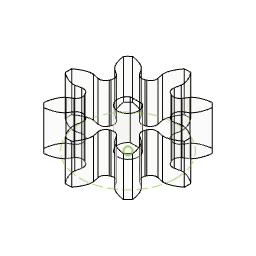
base driver spur gear v1 (Autodesk Fusion 360 archive; units mm, degrees)
design "base driver spur gear" references "Nema 17 groot", "Global Parameters"
description: Spur Gear; Module: 3.0; Num Teeth: 8; Pressure Angle: 20.0; Backlash: 0.00 mm
Autodesk Fusion 360 part; units mm, degrees
imported_body "Derived Base Feature1" makes body 1
other "Derived from Global Parameters v5"
sketch "Sketch1" plane through (0, 0, 0) normal (0, 0, 1) x (1, 0, 0) in component "Spur Gear (8 teeth)"
  circle A0 centre (0, 0) radius 8.3492
extrude "Extrude1" add sketch "Sketch1" along normal blind 10 separate body makes body 2 in component "Spur Gear (8 teeth)"
sketch "Sketch2" plane through (0, 0, 0) normal (0, 0, 1) x (1, 0, 0) in component "Spur Gear (8 teeth)"
  spline S0 degree 5 poles (11.0256, -2.3645) (11.0366, -2.3668) (11.0587, -2.3711) (11.092, -2.3763) (11.1367, -2.3808) (11.193, -2.3832) (11.2496, -2.3833) (11.3065, -2.3819) (11.3634, -2.3798) (11.4205, -2.3772) (11.4776, -2.3739) (11.5348, -2.3698) (11.5921, -2.3647) (11.6496, -2.3584) (11.7071, -2.3509) (11.7647, -2.3424) (11.8223, -2.3329) (11.88, -2.3226) (11.9378, -2.3117) (11.9955, -2.3) (12.0533, -2.2877) (12.111, -2.2747) (12.1688, -2.261) (12.2266, -2.2464) (12.2844, -2.2311) (12.3422, -2.2151) (12.4, -2.1984) (12.4578, -2.181) (12.5155, -2.163) (12.5732, -2.1444) (12.6309, -2.1252) (12.6886, -2.1053) (12.7462, -2.0848) (12.8038, -2.0636) (12.8613, -2.0419) (12.9188, -2.0195) (12.9762, -1.9965) (13.0336, -1.9729) (13.0909, -1.9488) (13.1481, -1.9241) (13.2052, -1.8988) (13.2623, -1.8729) (13.3193, -1.8465) (13.3763, -1.8195) (13.4331, -1.792) (13.4899, -1.7639) (13.5466, -1.7353) (13.6031, -1.7061) (13.6596, -1.6764) (13.716, -1.6461) (13.7723, -1.6153) (13.8284, -1.584) (13.8845, -1.5522) (13.9404, -1.5199) (13.9963, -1.487) (14.052, -1.4537) (14.1076, -1.4198) (14.163, -1.3854) (14.2183, -1.3506) (14.2735, -1.3152) (14.3286, -1.2793) (14.3836, -1.243) (14.4384, -1.2061) (14.493, -1.1688) (14.5475, -1.131) (14.6019, -1.0927) (14.6561, -1.054) (14.7102, -1.0147) (14.7641, -0.975) (14.8178, -0.9349) (14.8714, -0.8943) (14.9141, -0.8614) (14.9461, -0.8365) (14.9674, -0.8198) (14.978, -0.8115) knots 0 0 0 0 0 0 0.01428571 0.02857143 0.04285714 0.05714286 0.07142857 0.08571429 0.1 0.11428571 0.12857143 0.14285714 0.15714286 0.17142857 0.18571429 0.2 0.21428571 0.22857143 0.24285714 0.25714286 0.27142857 0.28571429 0.3 0.31428571 0.32857143 0.34285714 0.35714286 0.37142857 0.38571429 0.4 0.41428571 0.42857143 0.44285714 0.45714286 0.47142857 0.48571429 0.5 0.51428571 0.52857143 0.54285714 0.55714286 0.57142857 0.58571429 0.6 0.61428571 0.62857143 0.64285714 0.65714286 0.67142857 0.68571429 0.7 0.71428571 0.72857143 0.74285714 0.75714286 0.77142857 0.78571429 0.8 0.81428571 0.82857143 0.84285714 0.85714286 0.87142857 0.88571429 0.9 0.91428571 0.92857143 0.94285714 0.95714286 0.97142857 0.98571429 1 1 1 1 1 1
  spline S1 degree 5 poles (11.0256, 2.3645) (11.0366, 2.3668) (11.0587, 2.3711) (11.092, 2.3763) (11.1367, 2.3808) (11.193, 2.3832) (11.2496, 2.3833) (11.3065, 2.3819) (11.3634, 2.3798) (11.4205, 2.3772) (11.4776, 2.3739) (11.5348, 2.3698) (11.5921, 2.3647) (11.6496, 2.3584) (11.7071, 2.3509) (11.7647, 2.3424) (11.8223, 2.3329) (11.88, 2.3226) (11.9378, 2.3117) (11.9955, 2.3) (12.0533, 2.2877) (12.111, 2.2747) (12.1688, 2.261) (12.2266, 2.2464) (12.2844, 2.2311) (12.3422, 2.2151) (12.4, 2.1984) (12.4578, 2.181) (12.5155, 2.163) (12.5732, 2.1444) (12.6309, 2.1252) (12.6886, 2.1053) (12.7462, 2.0848) (12.8038, 2.0636) (12.8613, 2.0419) (12.9188, 2.0195) (12.9762, 1.9965) (13.0336, 1.9729) (13.0909, 1.9488) (13.1481, 1.9241) (13.2052, 1.8988) (13.2623, 1.8729) (13.3193, 1.8465) (13.3763, 1.8195) (13.4331, 1.792) (13.4899, 1.7639) (13.5466, 1.7353) (13.6031, 1.7061) (13.6596, 1.6764) (13.716, 1.6461) (13.7723, 1.6153) (13.8284, 1.584) (13.8845, 1.5522) (13.9404, 1.5199) (13.9963, 1.487) (14.052, 1.4537) (14.1076, 1.4198) (14.163, 1.3854) (14.2183, 1.3506) (14.2735, 1.3152) (14.3286, 1.2793) (14.3836, 1.243) (14.4384, 1.2061) (14.493, 1.1688) (14.5475, 1.131) (14.6019, 1.0927) (14.6561, 1.054) (14.7102, 1.0147) (14.7641, 0.975) (14.8178, 0.9349) (14.8714, 0.8943) (14.9141, 0.8614) (14.9461, 0.8365) (14.9674, 0.8198) (14.978, 0.8115) knots 0 0 0 0 0 0 0.01428571 0.02857143 0.04285714 0.05714286 0.07142857 0.08571429 0.1 0.11428571 0.12857143 0.14285714 0.15714286 0.17142857 0.18571429 0.2 0.21428571 0.22857143 0.24285714 0.25714286 0.27142857 0.28571429 0.3 0.31428571 0.32857143 0.34285714 0.35714286 0.37142857 0.38571429 0.4 0.41428571 0.42857143 0.44285714 0.45714286 0.47142857 0.48571429 0.5 0.51428571 0.52857143 0.54285714 0.55714286 0.57142857 0.58571429 0.6 0.61428571 0.62857143 0.64285714 0.65714286 0.67142857 0.68571429 0.7 0.71428571 0.72857143 0.74285714 0.75714286 0.77142857 0.78571429 0.8 0.81428571 0.82857143 0.84285714 0.85714286 0.87142857 0.88571429 0.9 0.91428571 0.92857143 0.94285714 0.95714286 0.97142857 0.98571429 1 1 1 1 1 1
  arc A0 (14.978, -0.8115) -> (14.978, 0.8115) centre (0, 0) ccw
  line L0 (8.1538, -1.7507) -> (11.0256, -2.3645)
  line L1 (8.1538, 1.7507) -> (11.0256, 2.3645)
  line L2 (8.1538, -1.7507) -> (8.1538, 1.7507)
  point P0 (11.2938, -2.3821)
  point P1 (11.5687, -2.3667)
  point P2 (11.8476, -2.3283)
  point P3 (12.1296, -2.2702)
  point P4 (12.4138, -2.1942)
  point P5 (12.6995, -2.1013)
  point P6 (12.9862, -1.9923)
  point P7 (13.2734, -1.8677)
  point P8 (13.5605, -1.728)
  point P9 (13.847, -1.5734)
  point P10 (14.1325, -1.4043)
  point P11 (14.4164, -1.2208)
  point P12 (14.6985, -1.0231)
  point P13 (11.2938, 2.3821)
  point P14 (11.5687, 2.3667)
  point P15 (11.8476, 2.3283)
  point P16 (12.1296, 2.2702)
  point P17 (12.4138, 2.1942)
  point P18 (12.6995, 2.1013)
  point P19 (12.9862, 1.9923)
  point P20 (13.2734, 1.8677)
  point P21 (13.5605, 1.728)
  point P22 (13.847, 1.5734)
  point P23 (14.1325, 1.4043)
  point P24 (14.4164, 1.2208)
  point P25 (14.6985, 1.0231)
extrude "Extrude2" add sketch "Sketch2" along normal blind 10 bodies 2 in component "Spur Gear (8 teeth)"
fillet "Fillet1" radius 1.5875 2 edges at (8.1632, -1.7527, 5) (8.1632, 1.7527, 5) on bodies 2 in component "Spur Gear (8 teeth)"
pattern_circular "C-Pattern1" count 8 over 360 about axis through (0, 0, 0) along (0, 0, 1) of "Extrude2", "Fillet1" in component "Spur Gear (8 teeth)"
sketch "Sketch3" plane through (0, 0, 0) normal (0, 0, 1) x (1, 0, 0) in component "Spur Gear (8 teeth)"
  circle A0 centre (0, 0) radius 12 construction
  dimension "dia_spurgear_2" = 24
  measures "dia_spurgear_2" diameter of A0
other "ExternalDerived2"
move_body "Move1" bodies 1 to x (1, 0, 0) y (0, 1, 0) z (0, 0, 1) at (0, 0, -20)
sketch "Sketch1 (2)" plane through (0, 0, 10) normal (0, 0, 1) x (-1, 0, 0)
  arc A0 (-7.6452, 3.3555) -> (-7.7787, 3.0333) centre (0, 0) ccw
  arc A1 (-9.5895, 2.0576) -> (-7.7787, 3.0333) centre (-9.2577, 3.61) ccw
  line L0 (-9.5895, 2.0576) -> (-11.0256, 2.3645)
  spline S0 degree 5 poles (-11.0256, 2.3645) (-11.0366, 2.3668) (-11.0587, 2.3711) (-11.092, 2.3763) (-11.1367, 2.3808) (-11.193, 2.3832) (-11.2496, 2.3833) (-11.3065, 2.3819) (-11.3634, 2.3798) (-11.4205, 2.3772) (-11.4776, 2.3739) (-11.5348, 2.3698) (-11.5921, 2.3647) (-11.6496, 2.3584) (-11.7071, 2.3509) (-11.7647, 2.3424) (-11.8223, 2.3329) (-11.88, 2.3226) (-11.9378, 2.3117) (-11.9955, 2.3) (-12.0533, 2.2877) (-12.111, 2.2747) (-12.1688, 2.261) (-12.2266, 2.2464) (-12.2844, 2.2311) (-12.3422, 2.2151) (-12.4, 2.1984) (-12.4578, 2.181) (-12.5155, 2.163) (-12.5732, 2.1444) (-12.6309, 2.1252) (-12.6886, 2.1053) (-12.7462, 2.0848) (-12.8038, 2.0636) (-12.8613, 2.0419) (-12.9188, 2.0195) (-12.9762, 1.9965) (-13.0336, 1.9729) (-13.0909, 1.9488) (-13.1481, 1.9241) (-13.2052, 1.8988) (-13.2623, 1.8729) (-13.3193, 1.8465) (-13.3763, 1.8195) (-13.4331, 1.792) (-13.4899, 1.7639) (-13.5466, 1.7353) (-13.6031, 1.7061) (-13.6596, 1.6764) (-13.716, 1.6461) (-13.7723, 1.6153) (-13.8284, 1.584) (-13.8845, 1.5522) (-13.9404, 1.5199) (-13.9963, 1.487) (-14.052, 1.4537) (-14.1076, 1.4198) (-14.163, 1.3854) (-14.2183, 1.3506) (-14.2735, 1.3152) (-14.3286, 1.2793) (-14.3836, 1.243) (-14.4384, 1.2061) (-14.493, 1.1688) (-14.5475, 1.131) (-14.6019, 1.0927) (-14.6561, 1.054) (-14.7102, 1.0147) (-14.7641, 0.975) (-14.8178, 0.9349) (-14.8714, 0.8943) (-14.9141, 0.8614) (-14.9461, 0.8365) (-14.9674, 0.8198) (-14.978, 0.8115) knots 0 0 0 0 0 0 0.01428571 0.02857143 0.04285714 0.05714286 0.07142857 0.08571429 0.1 0.11428571 0.12857143 0.14285714 0.15714286 0.17142857 0.18571429 0.2 0.21428571 0.22857143 0.24285714 0.25714286 0.27142857 0.28571429 0.3 0.31428571 0.32857143 0.34285714 0.35714286 0.37142857 0.38571429 0.4 0.41428571 0.42857143 0.44285714 0.45714286 0.47142857 0.48571429 0.5 0.51428571 0.52857143 0.54285714 0.55714286 0.57142857 0.58571429 0.6 0.61428571 0.62857143 0.64285714 0.65714286 0.67142857 0.68571429 0.7 0.71428571 0.72857143 0.74285714 0.75714286 0.77142857 0.78571429 0.8 0.81428571 0.82857143 0.84285714 0.85714286 0.87142857 0.88571429 0.9 0.91428571 0.92857143 0.94285714 0.95714286 0.97142857 0.98571429 1 1 1 1 1 1
  arc A2 (-14.978, 0.8115) -> (-14.978, -0.8115) centre (0, 0) ccw
  spline S1 degree 5 poles (-14.978, -0.8115) (-14.9674, -0.8198) (-14.9461, -0.8365) (-14.9141, -0.8614) (-14.8714, -0.8943) (-14.8178, -0.9349) (-14.7641, -0.975) (-14.7102, -1.0147) (-14.6561, -1.054) (-14.6019, -1.0927) (-14.5475, -1.131) (-14.493, -1.1688) (-14.4384, -1.2061) (-14.3836, -1.243) (-14.3286, -1.2793) (-14.2735, -1.3152) (-14.2183, -1.3506) (-14.163, -1.3854) (-14.1076, -1.4198) (-14.052, -1.4537) (-13.9963, -1.487) (-13.9404, -1.5199) (-13.8845, -1.5522) (-13.8284, -1.584) (-13.7723, -1.6153) (-13.716, -1.6461) (-13.6596, -1.6764) (-13.6031, -1.7061) (-13.5466, -1.7353) (-13.4899, -1.7639) (-13.4331, -1.792) (-13.3763, -1.8195) (-13.3193, -1.8465) (-13.2623, -1.8729) (-13.2052, -1.8988) (-13.1481, -1.9241) (-13.0909, -1.9488) (-13.0336, -1.9729) (-12.9762, -1.9965) (-12.9188, -2.0195) (-12.8613, -2.0419) (-12.8038, -2.0636) (-12.7462, -2.0848) (-12.6886, -2.1053) (-12.6309, -2.1252) (-12.5732, -2.1444) (-12.5155, -2.163) (-12.4578, -2.181) (-12.4, -2.1984) (-12.3422, -2.2151) (-12.2844, -2.2311) (-12.2266, -2.2464) (-12.1688, -2.261) (-12.111, -2.2747) (-12.0533, -2.2877) (-11.9955, -2.3) (-11.9378, -2.3117) (-11.88, -2.3226) (-11.8223, -2.3329) (-11.7647, -2.3424) (-11.7071, -2.3509) (-11.6496, -2.3584) (-11.5921, -2.3647) (-11.5348, -2.3698) (-11.4776, -2.3739) (-11.4205, -2.3772) (-11.3634, -2.3798) (-11.3065, -2.3819) (-11.2496, -2.3833) (-11.193, -2.3832) (-11.1367, -2.3808) (-11.092, -2.3763) (-11.0587, -2.3711) (-11.0366, -2.3668) (-11.0256, -2.3645) knots -1 -1 -1 -1 -1 -1 -0.98571429 -0.97142857 -0.95714286 -0.94285714 -0.92857143 -0.91428571 -0.9 -0.88571429 -0.87142857 -0.85714286 -0.84285714 -0.82857143 -0.81428571 -0.8 -0.78571429 -0.77142857 -0.75714286 -0.74285714 -0.72857143 -0.71428571 -0.7 -0.68571429 -0.67142857 -0.65714286 -0.64285714 -0.62857143 -0.61428571 -0.6 -0.58571429 -0.57142857 -0.55714286 -0.54285714 -0.52857143 -0.51428571 -0.5 -0.48571429 -0.47142857 -0.45714286 -0.44285714 -0.42857143 -0.41428571 -0.4 -0.38571429 -0.37142857 -0.35714286 -0.34285714 -0.32857143 -0.31428571 -0.3 -0.28571429 -0.27142857 -0.25714286 -0.24285714 -0.22857143 -0.21428571 -0.2 -0.18571429 -0.17142857 -0.15714286 -0.14285714 -0.12857143 -0.11428571 -0.1 -0.08571429 -0.07142857 -0.05714286 -0.04285714 -0.02857143 -0.01428571 0 0 0 0 0 0
  line L1 (-11.0256, -2.3645) -> (-9.5895, -2.0576)
  arc A3 (-7.7787, -3.0333) -> (-9.5895, -2.0576) centre (-9.2577, -3.61) ccw
  arc A4 (-8.2357, -5.3259) -> (-7.6452, -3.3555) centre (-9.0989, -3.9936) ccw
  line L2 (-8.2357, -5.3259) -> (-9.4682, -6.1244)
  spline S2 degree 5 poles (-9.4682, -6.1244) (-9.4777, -6.1305) (-9.4963, -6.1431) (-9.5235, -6.1629) (-9.5583, -6.1913) (-9.5998, -6.2295) (-9.6399, -6.2695) (-9.6792, -6.3106) (-9.718, -6.3524) (-9.7564, -6.3946) (-9.7945, -6.4373) (-9.8321, -6.4806) (-9.869, -6.5248) (-9.9051, -6.5698) (-9.9405, -6.6158) (-9.9752, -6.6626) (-10.0092, -6.7101) (-10.0428, -6.7581) (-10.0759, -6.8067) (-10.1085, -6.8557) (-10.1406, -6.9053) (-10.1723, -6.9553) (-10.2034, -7.0059) (-10.234, -7.0571) (-10.264, -7.1088) (-10.2936, -7.1609) (-10.3226, -7.2136) (-10.3512, -7.2667) (-10.3793, -7.3203) (-10.407, -7.3743) (-10.4341, -7.4287) (-10.4608, -7.4835) (-10.4871, -7.5388) (-10.5128, -7.5944) (-10.5381, -7.6505) (-10.5629, -7.707) (-10.5873, -7.7638) (-10.6112, -7.821) (-10.6346, -7.8786) (-10.6576, -7.9366) (-10.6802, -7.9949) (-10.7023, -8.0535) (-10.7239, -8.1125) (-10.7451, -8.1719) (-10.7658, -8.2315) (-10.7861, -8.2915) (-10.8059, -8.3519) (-10.8252, -8.4125) (-10.8442, -8.4734) (-10.8626, -8.5347) (-10.8807, -8.5962) (-10.8983, -8.6581) (-10.9154, -8.7202) (-10.9321, -8.7826) (-10.9483, -8.8454) (-10.9641, -8.9083) (-10.9795, -8.9716) (-10.9944, -9.0351) (-11.0089, -9.0989) (-11.0229, -9.1629) (-11.0365, -9.2272) (-11.0496, -9.2918) (-11.0623, -9.3566) (-11.0746, -9.4216) (-11.0864, -9.4869) (-11.0978, -9.5524) (-11.1087, -9.6182) (-11.1192, -9.6841) (-11.1292, -9.7503) (-11.1388, -9.8167) (-11.148, -9.8833) (-11.155, -9.9368) (-11.16, -9.977) (-11.1633, -10.0038) (-11.1649, -10.0173) knots 0 0 0 0 0 0 0.01428571 0.02857143 0.04285714 0.05714286 0.07142857 0.08571429 0.1 0.11428571 0.12857143 0.14285714 0.15714286 0.17142857 0.18571429 0.2 0.21428571 0.22857143 0.24285714 0.25714286 0.27142857 0.28571429 0.3 0.31428571 0.32857143 0.34285714 0.35714286 0.37142857 0.38571429 0.4 0.41428571 0.42857143 0.44285714 0.45714286 0.47142857 0.48571429 0.5 0.51428571 0.52857143 0.54285714 0.55714286 0.57142857 0.58571429 0.6 0.61428571 0.62857143 0.64285714 0.65714286 0.67142857 0.68571429 0.7 0.71428571 0.72857143 0.74285714 0.75714286 0.77142857 0.78571429 0.8 0.81428571 0.82857143 0.84285714 0.85714286 0.87142857 0.88571429 0.9 0.91428571 0.92857143 0.94285714 0.95714286 0.97142857 0.98571429 1 1 1 1 1 1
  arc A5 (-11.1649, -10.0173) -> (-10.0173, -11.1649) centre (0, 0) ccw
  spline S3 degree 5 poles (-10.0173, -11.1649) (-10.0038, -11.1633) (-9.977, -11.16) (-9.9368, -11.155) (-9.8833, -11.148) (-9.8167, -11.1388) (-9.7503, -11.1292) (-9.6841, -11.1192) (-9.6182, -11.1087) (-9.5524, -11.0978) (-9.4869, -11.0864) (-9.4216, -11.0746) (-9.3566, -11.0623) (-9.2918, -11.0496) (-9.2272, -11.0365) (-9.1629, -11.0229) (-9.0989, -11.0089) (-9.0351, -10.9944) (-8.9716, -10.9795) (-8.9083, -10.9641) (-8.8454, -10.9483) (-8.7826, -10.9321) (-8.7202, -10.9154) (-8.6581, -10.8983) (-8.5962, -10.8807) (-8.5347, -10.8626) (-8.4734, -10.8442) (-8.4125, -10.8252) (-8.3519, -10.8059) (-8.2915, -10.7861) (-8.2315, -10.7658) (-8.1719, -10.7451) (-8.1125, -10.7239) (-8.0535, -10.7023) (-7.9949, -10.6802) (-7.9366, -10.6576) (-7.8786, -10.6346) (-7.821, -10.6112) (-7.7638, -10.5873) (-7.707, -10.5629) (-7.6505, -10.5381) (-7.5944, -10.5128) (-7.5388, -10.4871) (-7.4835, -10.4608) (-7.4287, -10.4341) (-7.3743, -10.407) (-7.3203, -10.3793) (-7.2667, -10.3512) (-7.2136, -10.3226) (-7.1609, -10.2936) (-7.1088, -10.264) (-7.0571, -10.234) (-7.0059, -10.2034) (-6.9553, -10.1723) (-6.9053, -10.1406) (-6.8557, -10.1085) (-6.8067, -10.0759) (-6.7581, -10.0428) (-6.7101, -10.0092) (-6.6626, -9.9752) (-6.6158, -9.9405) (-6.5698, -9.9051) (-6.5248, -9.869) (-6.4806, -9.8321) (-6.4373, -9.7945) (-6.3946, -9.7564) (-6.3524, -9.718) (-6.3106, -9.6792) (-6.2695, -9.6399) (-6.2295, -9.5998) (-6.1913, -9.5583) (-6.1629, -9.5235) (-6.1431, -9.4963) (-6.1305, -9.4777) (-6.1244, -9.4682) knots -1 -1 -1 -1 -1 -1 -0.98571429 -0.97142857 -0.95714286 -0.94285714 -0.92857143 -0.91428571 -0.9 -0.88571429 -0.87142857 -0.85714286 -0.84285714 -0.82857143 -0.81428571 -0.8 -0.78571429 -0.77142857 -0.75714286 -0.74285714 -0.72857143 -0.71428571 -0.7 -0.68571429 -0.67142857 -0.65714286 -0.64285714 -0.62857143 -0.61428571 -0.6 -0.58571429 -0.57142857 -0.55714286 -0.54285714 -0.52857143 -0.51428571 -0.5 -0.48571429 -0.47142857 -0.45714286 -0.44285714 -0.42857143 -0.41428571 -0.4 -0.38571429 -0.37142857 -0.35714286 -0.34285714 -0.32857143 -0.31428571 -0.3 -0.28571429 -0.27142857 -0.25714286 -0.24285714 -0.22857143 -0.21428571 -0.2 -0.18571429 -0.17142857 -0.15714286 -0.14285714 -0.12857143 -0.11428571 -0.1 -0.08571429 -0.07142857 -0.05714286 -0.04285714 -0.02857143 -0.01428571 0 0 0 0 0 0
  line L3 (-6.1244, -9.4682) -> (-5.3259, -8.2357)
  arc A6 (-3.3555, -7.6452) -> (-5.3259, -8.2357) centre (-3.9936, -9.0989) ccw
  arc A7 (-2.0576, -9.5895) -> (-3.0333, -7.7787) centre (-3.61, -9.2577) ccw
  line L4 (-2.0576, -9.5895) -> (-2.3645, -11.0256)
  spline S4 degree 5 poles (-2.3645, -11.0256) (-2.3668, -11.0366) (-2.3711, -11.0587) (-2.3763, -11.092) (-2.3808, -11.1367) (-2.3832, -11.193) (-2.3833, -11.2496) (-2.3819, -11.3065) (-2.3798, -11.3634) (-2.3772, -11.4205) (-2.3739, -11.4776) (-2.3698, -11.5348) (-2.3647, -11.5921) (-2.3584, -11.6496) (-2.3509, -11.7071) (-2.3424, -11.7647) (-2.3329, -11.8223) (-2.3226, -11.88) (-2.3117, -11.9378) (-2.3, -11.9955) (-2.2877, -12.0533) (-2.2747, -12.111) (-2.261, -12.1688) (-2.2464, -12.2266) (-2.2311, -12.2844) (-2.2151, -12.3422) (-2.1984, -12.4) (-2.181, -12.4578) (-2.163, -12.5155) (-2.1444, -12.5732) (-2.1252, -12.6309) (-2.1053, -12.6886) (-2.0848, -12.7462) (-2.0636, -12.8038) (-2.0419, -12.8613) (-2.0195, -12.9188) (-1.9965, -12.9762) (-1.9729, -13.0336) (-1.9488, -13.0909) (-1.9241, -13.1481) (-1.8988, -13.2052) (-1.8729, -13.2623) (-1.8465, -13.3193) (-1.8195, -13.3763) (-1.792, -13.4331) (-1.7639, -13.4899) (-1.7353, -13.5466) (-1.7061, -13.6031) (-1.6764, -13.6596) (-1.6461, -13.716) (-1.6153, -13.7723) (-1.584, -13.8284) (-1.5522, -13.8845) (-1.5199, -13.9404) (-1.487, -13.9963) (-1.4537, -14.052) (-1.4198, -14.1076) (-1.3854, -14.163) (-1.3506, -14.2183) (-1.3152, -14.2735) (-1.2793, -14.3286) (-1.243, -14.3836) (-1.2061, -14.4384) (-1.1688, -14.493) (-1.131, -14.5475) (-1.0927, -14.6019) (-1.054, -14.6561) (-1.0147, -14.7102) (-0.975, -14.7641) (-0.9349, -14.8178) (-0.8943, -14.8714) (-0.8614, -14.9141) (-0.8365, -14.9461) (-0.8198, -14.9674) (-0.8115, -14.978) knots 0 0 0 0 0 0 0.01428571 0.02857143 0.04285714 0.05714286 0.07142857 0.08571429 0.1 0.11428571 0.12857143 0.14285714 0.15714286 0.17142857 0.18571429 0.2 0.21428571 0.22857143 0.24285714 0.25714286 0.27142857 0.28571429 0.3 0.31428571 0.32857143 0.34285714 0.35714286 0.37142857 0.38571429 0.4 0.41428571 0.42857143 0.44285714 0.45714286 0.47142857 0.48571429 0.5 0.51428571 0.52857143 0.54285714 0.55714286 0.57142857 0.58571429 0.6 0.61428571 0.62857143 0.64285714 0.65714286 0.67142857 0.68571429 0.7 0.71428571 0.72857143 0.74285714 0.75714286 0.77142857 0.78571429 0.8 0.81428571 0.82857143 0.84285714 0.85714286 0.87142857 0.88571429 0.9 0.91428571 0.92857143 0.94285714 0.95714286 0.97142857 0.98571429 1 1 1 1 1 1
  arc A8 (-0.8115, -14.978) -> (0.8115, -14.978) centre (0, 0) ccw
  spline S5 degree 5 poles (0.8115, -14.978) (0.8198, -14.9674) (0.8365, -14.9461) (0.8614, -14.9141) (0.8943, -14.8714) (0.9349, -14.8178) (0.975, -14.7641) (1.0147, -14.7102) (1.054, -14.6561) (1.0927, -14.6019) (1.131, -14.5475) (1.1688, -14.493) (1.2061, -14.4384) (1.243, -14.3836) (1.2793, -14.3286) (1.3152, -14.2735) (1.3506, -14.2183) (1.3854, -14.163) (1.4198, -14.1076) (1.4537, -14.052) (1.487, -13.9963) (1.5199, -13.9404) (1.5522, -13.8845) (1.584, -13.8284) (1.6153, -13.7723) (1.6461, -13.716) (1.6764, -13.6596) (1.7061, -13.6031) (1.7353, -13.5466) (1.7639, -13.4899) (1.792, -13.4331) (1.8195, -13.3763) (1.8465, -13.3193) (1.8729, -13.2623) (1.8988, -13.2052) (1.9241, -13.1481) (1.9488, -13.0909) (1.9729, -13.0336) (1.9965, -12.9762) (2.0195, -12.9188) (2.0419, -12.8613) (2.0636, -12.8038) (2.0848, -12.7462) (2.1053, -12.6886) (2.1252, -12.6309) (2.1444, -12.5732) (2.163, -12.5155) (2.181, -12.4578) (2.1984, -12.4) (2.2151, -12.3422) (2.2311, -12.2844) (2.2464, -12.2266) (2.261, -12.1688) (2.2747, -12.111) (2.2877, -12.0533) (2.3, -11.9955) (2.3117, -11.9378) (2.3226, -11.88) (2.3329, -11.8223) (2.3424, -11.7647) (2.3509, -11.7071) (2.3584, -11.6496) (2.3647, -11.5921) (2.3698, -11.5348) (2.3739, -11.4776) (2.3772, -11.4205) (2.3798, -11.3634) (2.3819, -11.3065) (2.3833, -11.2496) (2.3832, -11.193) (2.3808, -11.1367) (2.3763, -11.092) (2.3711, -11.0587) (2.3668, -11.0366) (2.3645, -11.0256) knots -1 -1 -1 -1 -1 -1 -0.98571429 -0.97142857 -0.95714286 -0.94285714 -0.92857143 -0.91428571 -0.9 -0.88571429 -0.87142857 -0.85714286 -0.84285714 -0.82857143 -0.81428571 -0.8 -0.78571429 -0.77142857 -0.75714286 -0.74285714 -0.72857143 -0.71428571 -0.7 -0.68571429 -0.67142857 -0.65714286 -0.64285714 -0.62857143 -0.61428571 -0.6 -0.58571429 -0.57142857 -0.55714286 -0.54285714 -0.52857143 -0.51428571 -0.5 -0.48571429 -0.47142857 -0.45714286 -0.44285714 -0.42857143 -0.41428571 -0.4 -0.38571429 -0.37142857 -0.35714286 -0.34285714 -0.32857143 -0.31428571 -0.3 -0.28571429 -0.27142857 -0.25714286 -0.24285714 -0.22857143 -0.21428571 -0.2 -0.18571429 -0.17142857 -0.15714286 -0.14285714 -0.12857143 -0.11428571 -0.1 -0.08571429 -0.07142857 -0.05714286 -0.04285714 -0.02857143 -0.01428571 0 0 0 0 0 0
  line L5 (2.3645, -11.0256) -> (2.0576, -9.5895)
  arc A9 (3.0333, -7.7787) -> (2.0576, -9.5895) centre (3.61, -9.2577) ccw
  arc A10 (5.3259, -8.2357) -> (3.3555, -7.6452) centre (3.9936, -9.0989) ccw
  line L6 (5.3259, -8.2357) -> (6.1244, -9.4682)
  spline S6 degree 5 poles (6.1244, -9.4682) (6.1305, -9.4777) (6.1431, -9.4963) (6.1629, -9.5235) (6.1913, -9.5583) (6.2295, -9.5998) (6.2695, -9.6399) (6.3106, -9.6792) (6.3524, -9.718) (6.3946, -9.7564) (6.4373, -9.7945) (6.4806, -9.8321) (6.5248, -9.869) (6.5698, -9.9051) (6.6158, -9.9405) (6.6626, -9.9752) (6.7101, -10.0092) (6.7581, -10.0428) (6.8067, -10.0759) (6.8557, -10.1085) (6.9053, -10.1406) (6.9553, -10.1723) (7.0059, -10.2034) (7.0571, -10.234) (7.1088, -10.264) (7.1609, -10.2936) (7.2136, -10.3226) (7.2667, -10.3512) (7.3203, -10.3793) (7.3743, -10.407) (7.4287, -10.4341) (7.4835, -10.4608) (7.5388, -10.4871) (7.5944, -10.5128) (7.6505, -10.5381) (7.707, -10.5629) (7.7638, -10.5873) (7.821, -10.6112) (7.8786, -10.6346) (7.9366, -10.6576) (7.9949, -10.6802) (8.0535, -10.7023) (8.1125, -10.7239) (8.1719, -10.7451) (8.2315, -10.7658) (8.2915, -10.7861) (8.3519, -10.8059) (8.4125, -10.8252) (8.4734, -10.8442) (8.5347, -10.8626) (8.5962, -10.8807) (8.6581, -10.8983) (8.7202, -10.9154) (8.7826, -10.9321) (8.8454, -10.9483) (8.9083, -10.9641) (8.9716, -10.9795) (9.0351, -10.9944) (9.0989, -11.0089) (9.1629, -11.0229) (9.2272, -11.0365) (9.2918, -11.0496) (9.3566, -11.0623) (9.4216, -11.0746) (9.4869, -11.0864) (9.5524, -11.0978) (9.6182, -11.1087) (9.6841, -11.1192) (9.7503, -11.1292) (9.8167, -11.1388) (9.8833, -11.148) (9.9368, -11.155) (9.977, -11.16) (10.0038, -11.1633) (10.0173, -11.1649) knots 0 0 0 0 0 0 0.01428571 0.02857143 0.04285714 0.05714286 0.07142857 0.08571429 0.1 0.11428571 0.12857143 0.14285714 0.15714286 0.17142857 0.18571429 0.2 0.21428571 0.22857143 0.24285714 0.25714286 0.27142857 0.28571429 0.3 0.31428571 0.32857143 0.34285714 0.35714286 0.37142857 0.38571429 0.4 0.41428571 0.42857143 0.44285714 0.45714286 0.47142857 0.48571429 0.5 0.51428571 0.52857143 0.54285714 0.55714286 0.57142857 0.58571429 0.6 0.61428571 0.62857143 0.64285714 0.65714286 0.67142857 0.68571429 0.7 0.71428571 0.72857143 0.74285714 0.75714286 0.77142857 0.78571429 0.8 0.81428571 0.82857143 0.84285714 0.85714286 0.87142857 0.88571429 0.9 0.91428571 0.92857143 0.94285714 0.95714286 0.97142857 0.98571429 1 1 1 1 1 1
  arc A11 (10.0173, -11.1649) -> (11.1649, -10.0173) centre (0, 0) ccw
  spline S7 degree 5 poles (11.1649, -10.0173) (11.1633, -10.0038) (11.16, -9.977) (11.155, -9.9368) (11.148, -9.8833) (11.1388, -9.8167) (11.1292, -9.7503) (11.1192, -9.6841) (11.1087, -9.6182) (11.0978, -9.5524) (11.0864, -9.4869) (11.0746, -9.4216) (11.0623, -9.3566) (11.0496, -9.2918) (11.0365, -9.2272) (11.0229, -9.1629) (11.0089, -9.0989) (10.9944, -9.0351) (10.9795, -8.9716) (10.9641, -8.9083) (10.9483, -8.8454) (10.9321, -8.7826) (10.9154, -8.7202) (10.8983, -8.6581) (10.8807, -8.5962) (10.8626, -8.5347) (10.8442, -8.4734) (10.8252, -8.4125) (10.8059, -8.3519) (10.7861, -8.2915) (10.7658, -8.2315) (10.7451, -8.1719) (10.7239, -8.1125) (10.7023, -8.0535) (10.6802, -7.9949) (10.6576, -7.9366) (10.6346, -7.8786) (10.6112, -7.821) (10.5873, -7.7638) (10.5629, -7.707) (10.5381, -7.6505) (10.5128, -7.5944) (10.4871, -7.5388) (10.4608, -7.4835) (10.4341, -7.4287) (10.407, -7.3743) (10.3793, -7.3203) (10.3512, -7.2667) (10.3226, -7.2136) (10.2936, -7.1609) (10.264, -7.1088) (10.234, -7.0571) (10.2034, -7.0059) (10.1723, -6.9553) (10.1406, -6.9053) (10.1085, -6.8557) (10.0759, -6.8067) (10.0428, -6.7581) (10.0092, -6.7101) (9.9752, -6.6626) (9.9405, -6.6158) (9.9051, -6.5698) (9.869, -6.5248) (9.8321, -6.4806) (9.7945, -6.4373) (9.7564, -6.3946) (9.718, -6.3524) (9.6792, -6.3106) (9.6399, -6.2695) (9.5998, -6.2295) (9.5583, -6.1913) (9.5235, -6.1629) (9.4963, -6.1431) (9.4777, -6.1305) (9.4682, -6.1244) knots -1 -1 -1 -1 -1 -1 -0.98571429 -0.97142857 -0.95714286 -0.94285714 -0.92857143 -0.91428571 -0.9 -0.88571429 -0.87142857 -0.85714286 -0.84285714 -0.82857143 -0.81428571 -0.8 -0.78571429 -0.77142857 -0.75714286 -0.74285714 -0.72857143 -0.71428571 -0.7 -0.68571429 -0.67142857 -0.65714286 -0.64285714 -0.62857143 -0.61428571 -0.6 -0.58571429 -0.57142857 -0.55714286 -0.54285714 -0.52857143 -0.51428571 -0.5 -0.48571429 -0.47142857 -0.45714286 -0.44285714 -0.42857143 -0.41428571 -0.4 -0.38571429 -0.37142857 -0.35714286 -0.34285714 -0.32857143 -0.31428571 -0.3 -0.28571429 -0.27142857 -0.25714286 -0.24285714 -0.22857143 -0.21428571 -0.2 -0.18571429 -0.17142857 -0.15714286 -0.14285714 -0.12857143 -0.11428571 -0.1 -0.08571429 -0.07142857 -0.05714286 -0.04285714 -0.02857143 -0.01428571 0 0 0 0 0 0
  line L7 (9.4682, -6.1244) -> (8.2357, -5.3259)
  arc A12 (7.6452, -3.3555) -> (8.2357, -5.3259) centre (9.0989, -3.9936) ccw
  arc A13 (9.5895, -2.0576) -> (7.7787, -3.0333) centre (9.2577, -3.61) ccw
  line L8 (9.5895, -2.0576) -> (11.0256, -2.3645)
  spline S8 degree 5 poles (11.0256, -2.3645) (11.0366, -2.3668) (11.0587, -2.3711) (11.092, -2.3763) (11.1367, -2.3808) (11.193, -2.3832) (11.2496, -2.3833) (11.3065, -2.3819) (11.3634, -2.3798) (11.4205, -2.3772) (11.4776, -2.3739) (11.5348, -2.3698) (11.5921, -2.3647) (11.6496, -2.3584) (11.7071, -2.3509) (11.7647, -2.3424) (11.8223, -2.3329) (11.88, -2.3226) (11.9378, -2.3117) (11.9955, -2.3) (12.0533, -2.2877) (12.111, -2.2747) (12.1688, -2.261) (12.2266, -2.2464) (12.2844, -2.2311) (12.3422, -2.2151) (12.4, -2.1984) (12.4578, -2.181) (12.5155, -2.163) (12.5732, -2.1444) (12.6309, -2.1252) (12.6886, -2.1053) (12.7462, -2.0848) (12.8038, -2.0636) (12.8613, -2.0419) (12.9188, -2.0195) (12.9762, -1.9965) (13.0336, -1.9729) (13.0909, -1.9488) (13.1481, -1.9241) (13.2052, -1.8988) (13.2623, -1.8729) (13.3193, -1.8465) (13.3763, -1.8195) (13.4331, -1.792) (13.4899, -1.7639) (13.5466, -1.7353) (13.6031, -1.7061) (13.6596, -1.6764) (13.716, -1.6461) (13.7723, -1.6153) (13.8284, -1.584) (13.8845, -1.5522) (13.9404, -1.5199) (13.9963, -1.487) (14.052, -1.4537) (14.1076, -1.4198) (14.163, -1.3854) (14.2183, -1.3506) (14.2735, -1.3152) (14.3286, -1.2793) (14.3836, -1.243) (14.4384, -1.2061) (14.493, -1.1688) (14.5475, -1.131) (14.6019, -1.0927) (14.6561, -1.054) (14.7102, -1.0147) (14.7641, -0.975) (14.8178, -0.9349) (14.8714, -0.8943) (14.9141, -0.8614) (14.9461, -0.8365) (14.9674, -0.8198) (14.978, -0.8115) knots 0 0 0 0 0 0 0.01428571 0.02857143 0.04285714 0.05714286 0.07142857 0.08571429 0.1 0.11428571 0.12857143 0.14285714 0.15714286 0.17142857 0.18571429 0.2 0.21428571 0.22857143 0.24285714 0.25714286 0.27142857 0.28571429 0.3 0.31428571 0.32857143 0.34285714 0.35714286 0.37142857 0.38571429 0.4 0.41428571 0.42857143 0.44285714 0.45714286 0.47142857 0.48571429 0.5 0.51428571 0.52857143 0.54285714 0.55714286 0.57142857 0.58571429 0.6 0.61428571 0.62857143 0.64285714 0.65714286 0.67142857 0.68571429 0.7 0.71428571 0.72857143 0.74285714 0.75714286 0.77142857 0.78571429 0.8 0.81428571 0.82857143 0.84285714 0.85714286 0.87142857 0.88571429 0.9 0.91428571 0.92857143 0.94285714 0.95714286 0.97142857 0.98571429 1 1 1 1 1 1
  arc A14 (14.978, -0.8115) -> (14.978, 0.8115) centre (0, 0) ccw
  spline S9 degree 5 poles (14.978, 0.8115) (14.9674, 0.8198) (14.9461, 0.8365) (14.9141, 0.8614) (14.8714, 0.8943) (14.8178, 0.9349) (14.7641, 0.975) (14.7102, 1.0147) (14.6561, 1.054) (14.6019, 1.0927) (14.5475, 1.131) (14.493, 1.1688) (14.4384, 1.2061) (14.3836, 1.243) (14.3286, 1.2793) (14.2735, 1.3152) (14.2183, 1.3506) (14.163, 1.3854) (14.1076, 1.4198) (14.052, 1.4537) (13.9963, 1.487) (13.9404, 1.5199) (13.8845, 1.5522) (13.8284, 1.584) (13.7723, 1.6153) (13.716, 1.6461) (13.6596, 1.6764) (13.6031, 1.7061) (13.5466, 1.7353) (13.4899, 1.7639) (13.4331, 1.792) (13.3763, 1.8195) (13.3193, 1.8465) (13.2623, 1.8729) (13.2052, 1.8988) (13.1481, 1.9241) (13.0909, 1.9488) (13.0336, 1.9729) (12.9762, 1.9965) (12.9188, 2.0195) (12.8613, 2.0419) (12.8038, 2.0636) (12.7462, 2.0848) (12.6886, 2.1053) (12.6309, 2.1252) (12.5732, 2.1444) (12.5155, 2.163) (12.4578, 2.181) (12.4, 2.1984) (12.3422, 2.2151) (12.2844, 2.2311) (12.2266, 2.2464) (12.1688, 2.261) (12.111, 2.2747) (12.0533, 2.2877) (11.9955, 2.3) (11.9378, 2.3117) (11.88, 2.3226) (11.8223, 2.3329) (11.7647, 2.3424) (11.7071, 2.3509) (11.6496, 2.3584) (11.5921, 2.3647) (11.5348, 2.3698) (11.4776, 2.3739) (11.4205, 2.3772) (11.3634, 2.3798) (11.3065, 2.3819) (11.2496, 2.3833) (11.193, 2.3832) (11.1367, 2.3808) (11.092, 2.3763) (11.0587, 2.3711) (11.0366, 2.3668) (11.0256, 2.3645) knots -1 -1 -1 -1 -1 -1 -0.98571429 -0.97142857 -0.95714286 -0.94285714 -0.92857143 -0.91428571 -0.9 -0.88571429 -0.87142857 -0.85714286 -0.84285714 -0.82857143 -0.81428571 -0.8 -0.78571429 -0.77142857 -0.75714286 -0.74285714 -0.72857143 -0.71428571 -0.7 -0.68571429 -0.67142857 -0.65714286 -0.64285714 -0.62857143 -0.61428571 -0.6 -0.58571429 -0.57142857 -0.55714286 -0.54285714 -0.52857143 -0.51428571 -0.5 -0.48571429 -0.47142857 -0.45714286 -0.44285714 -0.42857143 -0.41428571 -0.4 -0.38571429 -0.37142857 -0.35714286 -0.34285714 -0.32857143 -0.31428571 -0.3 -0.28571429 -0.27142857 -0.25714286 -0.24285714 -0.22857143 -0.21428571 -0.2 -0.18571429 -0.17142857 -0.15714286 -0.14285714 -0.12857143 -0.11428571 -0.1 -0.08571429 -0.07142857 -0.05714286 -0.04285714 -0.02857143 -0.01428571 0 0 0 0 0 0
  line L9 (11.0256, 2.3645) -> (9.5895, 2.0576)
  arc A15 (7.7787, 3.0333) -> (9.5895, 2.0576) centre (9.2577, 3.61) ccw
  arc A16 (8.2357, 5.3259) -> (7.6452, 3.3555) centre (9.0989, 3.9936) ccw
  line L10 (8.2357, 5.3259) -> (9.4682, 6.1244)
  spline S10 degree 5 poles (9.4682, 6.1244) (9.4777, 6.1305) (9.4963, 6.1431) (9.5235, 6.1629) (9.5583, 6.1913) (9.5998, 6.2295) (9.6399, 6.2695) (9.6792, 6.3106) (9.718, 6.3524) (9.7564, 6.3946) (9.7945, 6.4373) (9.8321, 6.4806) (9.869, 6.5248) (9.9051, 6.5698) (9.9405, 6.6158) (9.9752, 6.6626) (10.0092, 6.7101) (10.0428, 6.7581) (10.0759, 6.8067) (10.1085, 6.8557) (10.1406, 6.9053) (10.1723, 6.9553) (10.2034, 7.0059) (10.234, 7.0571) (10.264, 7.1088) (10.2936, 7.1609) (10.3226, 7.2136) (10.3512, 7.2667) (10.3793, 7.3203) (10.407, 7.3743) (10.4341, 7.4287) (10.4608, 7.4835) (10.4871, 7.5388) (10.5128, 7.5944) (10.5381, 7.6505) (10.5629, 7.707) (10.5873, 7.7638) (10.6112, 7.821) (10.6346, 7.8786) (10.6576, 7.9366) (10.6802, 7.9949) (10.7023, 8.0535) (10.7239, 8.1125) (10.7451, 8.1719) (10.7658, 8.2315) (10.7861, 8.2915) (10.8059, 8.3519) (10.8252, 8.4125) (10.8442, 8.4734) (10.8626, 8.5347) (10.8807, 8.5962) (10.8983, 8.6581) (10.9154, 8.7202) (10.9321, 8.7826) (10.9483, 8.8454) (10.9641, 8.9083) (10.9795, 8.9716) (10.9944, 9.0351) (11.0089, 9.0989) (11.0229, 9.1629) (11.0365, 9.2272) (11.0496, 9.2918) (11.0623, 9.3566) (11.0746, 9.4216) (11.0864, 9.4869) (11.0978, 9.5524) (11.1087, 9.6182) (11.1192, 9.6841) (11.1292, 9.7503) (11.1388, 9.8167) (11.148, 9.8833) (11.155, 9.9368) (11.16, 9.977) (11.1633, 10.0038) (11.1649, 10.0173) knots 0 0 0 0 0 0 0.01428571 0.02857143 0.04285714 0.05714286 0.07142857 0.08571429 0.1 0.11428571 0.12857143 0.14285714 0.15714286 0.17142857 0.18571429 0.2 0.21428571 0.22857143 0.24285714 0.25714286 0.27142857 0.28571429 0.3 0.31428571 0.32857143 0.34285714 0.35714286 0.37142857 0.38571429 0.4 0.41428571 0.42857143 0.44285714 0.45714286 0.47142857 0.48571429 0.5 0.51428571 0.52857143 0.54285714 0.55714286 0.57142857 0.58571429 0.6 0.61428571 0.62857143 0.64285714 0.65714286 0.67142857 0.68571429 0.7 0.71428571 0.72857143 0.74285714 0.75714286 0.77142857 0.78571429 0.8 0.81428571 0.82857143 0.84285714 0.85714286 0.87142857 0.88571429 0.9 0.91428571 0.92857143 0.94285714 0.95714286 0.97142857 0.98571429 1 1 1 1 1 1
  arc A17 (11.1649, 10.0173) -> (10.0173, 11.1649) centre (0, 0) ccw
  spline S11 degree 5 poles (10.0173, 11.1649) (10.0038, 11.1633) (9.977, 11.16) (9.9368, 11.155) (9.8833, 11.148) (9.8167, 11.1388) (9.7503, 11.1292) (9.6841, 11.1192) (9.6182, 11.1087) (9.5524, 11.0978) (9.4869, 11.0864) (9.4216, 11.0746) (9.3566, 11.0623) (9.2918, 11.0496) (9.2272, 11.0365) (9.1629, 11.0229) (9.0989, 11.0089) (9.0351, 10.9944) (8.9716, 10.9795) (8.9083, 10.9641) (8.8454, 10.9483) (8.7826, 10.9321) (8.7202, 10.9154) (8.6581, 10.8983) (8.5962, 10.8807) (8.5347, 10.8626) (8.4734, 10.8442) (8.4125, 10.8252) (8.3519, 10.8059) (8.2915, 10.7861) (8.2315, 10.7658) (8.1719, 10.7451) (8.1125, 10.7239) (8.0535, 10.7023) (7.9949, 10.6802) (7.9366, 10.6576) (7.8786, 10.6346) (7.821, 10.6112) (7.7638, 10.5873) (7.707, 10.5629) (7.6505, 10.5381) (7.5944, 10.5128) (7.5388, 10.4871) (7.4835, 10.4608) (7.4287, 10.4341) (7.3743, 10.407) (7.3203, 10.3793) (7.2667, 10.3512) (7.2136, 10.3226) (7.1609, 10.2936) (7.1088, 10.264) (7.0571, 10.234) (7.0059, 10.2034) (6.9553, 10.1723) (6.9053, 10.1406) (6.8557, 10.1085) (6.8067, 10.0759) (6.7581, 10.0428) (6.7101, 10.0092) (6.6626, 9.9752) (6.6158, 9.9405) (6.5698, 9.9051) (6.5248, 9.869) (6.4806, 9.8321) (6.4373, 9.7945) (6.3946, 9.7564) (6.3524, 9.718) (6.3106, 9.6792) (6.2695, 9.6399) (6.2295, 9.5998) (6.1913, 9.5583) (6.1629, 9.5235) (6.1431, 9.4963) (6.1305, 9.4777) (6.1244, 9.4682) knots -1 -1 -1 -1 -1 -1 -0.98571429 -0.97142857 -0.95714286 -0.94285714 -0.92857143 -0.91428571 -0.9 -0.88571429 -0.87142857 -0.85714286 -0.84285714 -0.82857143 -0.81428571 -0.8 -0.78571429 -0.77142857 -0.75714286 -0.74285714 -0.72857143 -0.71428571 -0.7 -0.68571429 -0.67142857 -0.65714286 -0.64285714 -0.62857143 -0.61428571 -0.6 -0.58571429 -0.57142857 -0.55714286 -0.54285714 -0.52857143 -0.51428571 -0.5 -0.48571429 -0.47142857 -0.45714286 -0.44285714 -0.42857143 -0.41428571 -0.4 -0.38571429 -0.37142857 -0.35714286 -0.34285714 -0.32857143 -0.31428571 -0.3 -0.28571429 -0.27142857 -0.25714286 -0.24285714 -0.22857143 -0.21428571 -0.2 -0.18571429 -0.17142857 -0.15714286 -0.14285714 -0.12857143 -0.11428571 -0.1 -0.08571429 -0.07142857 -0.05714286 -0.04285714 -0.02857143 -0.01428571 0 0 0 0 0 0
  line L11 (6.1244, 9.4682) -> (5.3259, 8.2357)
  arc A18 (3.3555, 7.6452) -> (5.3259, 8.2357) centre (3.9936, 9.0989) ccw
  arc A19 (2.0576, 9.5895) -> (3.0333, 7.7787) centre (3.61, 9.2577) ccw
  line L12 (2.0576, 9.5895) -> (2.3645, 11.0256)
  spline S12 degree 5 poles (2.3645, 11.0256) (2.3668, 11.0366) (2.3711, 11.0587) (2.3763, 11.092) (2.3808, 11.1367) (2.3832, 11.193) (2.3833, 11.2496) (2.3819, 11.3065) (2.3798, 11.3634) (2.3772, 11.4205) (2.3739, 11.4776) (2.3698, 11.5348) (2.3647, 11.5921) (2.3584, 11.6496) (2.3509, 11.7071) (2.3424, 11.7647) (2.3329, 11.8223) (2.3226, 11.88) (2.3117, 11.9378) (2.3, 11.9955) (2.2877, 12.0533) (2.2747, 12.111) (2.261, 12.1688) (2.2464, 12.2266) (2.2311, 12.2844) (2.2151, 12.3422) (2.1984, 12.4) (2.181, 12.4578) (2.163, 12.5155) (2.1444, 12.5732) (2.1252, 12.6309) (2.1053, 12.6886) (2.0848, 12.7462) (2.0636, 12.8038) (2.0419, 12.8613) (2.0195, 12.9188) (1.9965, 12.9762) (1.9729, 13.0336) (1.9488, 13.0909) (1.9241, 13.1481) (1.8988, 13.2052) (1.8729, 13.2623) (1.8465, 13.3193) (1.8195, 13.3763) (1.792, 13.4331) (1.7639, 13.4899) (1.7353, 13.5466) (1.7061, 13.6031) (1.6764, 13.6596) (1.6461, 13.716) (1.6153, 13.7723) (1.584, 13.8284) (1.5522, 13.8845) (1.5199, 13.9404) (1.487, 13.9963) (1.4537, 14.052) (1.4198, 14.1076) (1.3854, 14.163) (1.3506, 14.2183) (1.3152, 14.2735) (1.2793, 14.3286) (1.243, 14.3836) (1.2061, 14.4384) (1.1688, 14.493) (1.131, 14.5475) (1.0927, 14.6019) (1.054, 14.6561) (1.0147, 14.7102) (0.975, 14.7641) (0.9349, 14.8178) (0.8943, 14.8714) (0.8614, 14.9141) (0.8365, 14.9461) (0.8198, 14.9674) (0.8115, 14.978) knots 0 0 0 0 0 0 0.01428571 0.02857143 0.04285714 0.05714286 0.07142857 0.08571429 0.1 0.11428571 0.12857143 0.14285714 0.15714286 0.17142857 0.18571429 0.2 0.21428571 0.22857143 0.24285714 0.25714286 0.27142857 0.28571429 0.3 0.31428571 0.32857143 0.34285714 0.35714286 0.37142857 0.38571429 0.4 0.41428571 0.42857143 0.44285714 0.45714286 0.47142857 0.48571429 0.5 0.51428571 0.52857143 0.54285714 0.55714286 0.57142857 0.58571429 0.6 0.61428571 0.62857143 0.64285714 0.65714286 0.67142857 0.68571429 0.7 0.71428571 0.72857143 0.74285714 0.75714286 0.77142857 0.78571429 0.8 0.81428571 0.82857143 0.84285714 0.85714286 0.87142857 0.88571429 0.9 0.91428571 0.92857143 0.94285714 0.95714286 0.97142857 0.98571429 1 1 1 1 1 1
  arc A20 (0.8115, 14.978) -> (-0.8115, 14.978) centre (0, 0) ccw
  spline S13 degree 5 poles (-0.8115, 14.978) (-0.8198, 14.9674) (-0.8365, 14.9461) (-0.8614, 14.9141) (-0.8943, 14.8714) (-0.9349, 14.8178) (-0.975, 14.7641) (-1.0147, 14.7102) (-1.054, 14.6561) (-1.0927, 14.6019) (-1.131, 14.5475) (-1.1688, 14.493) (-1.2061, 14.4384) (-1.243, 14.3836) (-1.2793, 14.3286) (-1.3152, 14.2735) (-1.3506, 14.2183) (-1.3854, 14.163) (-1.4198, 14.1076) (-1.4537, 14.052) (-1.487, 13.9963) (-1.5199, 13.9404) (-1.5522, 13.8845) (-1.584, 13.8284) (-1.6153, 13.7723) (-1.6461, 13.716) (-1.6764, 13.6596) (-1.7061, 13.6031) (-1.7353, 13.5466) (-1.7639, 13.4899) (-1.792, 13.4331) (-1.8195, 13.3763) (-1.8465, 13.3193) (-1.8729, 13.2623) (-1.8988, 13.2052) (-1.9241, 13.1481) (-1.9488, 13.0909) (-1.9729, 13.0336) (-1.9965, 12.9762) (-2.0195, 12.9188) (-2.0419, 12.8613) (-2.0636, 12.8038) (-2.0848, 12.7462) (-2.1053, 12.6886) (-2.1252, 12.6309) (-2.1444, 12.5732) (-2.163, 12.5155) (-2.181, 12.4578) (-2.1984, 12.4) (-2.2151, 12.3422) (-2.2311, 12.2844) (-2.2464, 12.2266) (-2.261, 12.1688) (-2.2747, 12.111) (-2.2877, 12.0533) (-2.3, 11.9955) (-2.3117, 11.9378) (-2.3226, 11.88) (-2.3329, 11.8223) (-2.3424, 11.7647) (-2.3509, 11.7071) (-2.3584, 11.6496) (-2.3647, 11.5921) (-2.3698, 11.5348) (-2.3739, 11.4776) (-2.3772, 11.4205) (-2.3798, 11.3634) (-2.3819, 11.3065) (-2.3833, 11.2496) (-2.3832, 11.193) (-2.3808, 11.1367) (-2.3763, 11.092) (-2.3711, 11.0587) (-2.3668, 11.0366) (-2.3645, 11.0256) knots -1 -1 -1 -1 -1 -1 -0.98571429 -0.97142857 -0.95714286 -0.94285714 -0.92857143 -0.91428571 -0.9 -0.88571429 -0.87142857 -0.85714286 -0.84285714 -0.82857143 -0.81428571 -0.8 -0.78571429 -0.77142857 -0.75714286 -0.74285714 -0.72857143 -0.71428571 -0.7 -0.68571429 -0.67142857 -0.65714286 -0.64285714 -0.62857143 -0.61428571 -0.6 -0.58571429 -0.57142857 -0.55714286 -0.54285714 -0.52857143 -0.51428571 -0.5 -0.48571429 -0.47142857 -0.45714286 -0.44285714 -0.42857143 -0.41428571 -0.4 -0.38571429 -0.37142857 -0.35714286 -0.34285714 -0.32857143 -0.31428571 -0.3 -0.28571429 -0.27142857 -0.25714286 -0.24285714 -0.22857143 -0.21428571 -0.2 -0.18571429 -0.17142857 -0.15714286 -0.14285714 -0.12857143 -0.11428571 -0.1 -0.08571429 -0.07142857 -0.05714286 -0.04285714 -0.02857143 -0.01428571 0 0 0 0 0 0
  line L13 (-2.3645, 11.0256) -> (-2.0576, 9.5895)
  arc A21 (-3.0333, 7.7787) -> (-2.0576, 9.5895) centre (-3.61, 9.2577) ccw
  arc A22 (-5.3259, 8.2357) -> (-3.3555, 7.6452) centre (-3.9936, 9.0989) ccw
  line L14 (-5.3259, 8.2357) -> (-6.1244, 9.4682)
  spline S14 degree 5 poles (-6.1244, 9.4682) (-6.1305, 9.4777) (-6.1431, 9.4963) (-6.1629, 9.5235) (-6.1913, 9.5583) (-6.2295, 9.5998) (-6.2695, 9.6399) (-6.3106, 9.6792) (-6.3524, 9.718) (-6.3946, 9.7564) (-6.4373, 9.7945) (-6.4806, 9.8321) (-6.5248, 9.869) (-6.5698, 9.9051) (-6.6158, 9.9405) (-6.6626, 9.9752) (-6.7101, 10.0092) (-6.7581, 10.0428) (-6.8067, 10.0759) (-6.8557, 10.1085) (-6.9053, 10.1406) (-6.9553, 10.1723) (-7.0059, 10.2034) (-7.0571, 10.234) (-7.1088, 10.264) (-7.1609, 10.2936) (-7.2136, 10.3226) (-7.2667, 10.3512) (-7.3203, 10.3793) (-7.3743, 10.407) (-7.4287, 10.4341) (-7.4835, 10.4608) (-7.5388, 10.4871) (-7.5944, 10.5128) (-7.6505, 10.5381) (-7.707, 10.5629) (-7.7638, 10.5873) (-7.821, 10.6112) (-7.8786, 10.6346) (-7.9366, 10.6576) (-7.9949, 10.6802) (-8.0535, 10.7023) (-8.1125, 10.7239) (-8.1719, 10.7451) (-8.2315, 10.7658) (-8.2915, 10.7861) (-8.3519, 10.8059) (-8.4125, 10.8252) (-8.4734, 10.8442) (-8.5347, 10.8626) (-8.5962, 10.8807) (-8.6581, 10.8983) (-8.7202, 10.9154) (-8.7826, 10.9321) (-8.8454, 10.9483) (-8.9083, 10.9641) (-8.9716, 10.9795) (-9.0351, 10.9944) (-9.0989, 11.0089) (-9.1629, 11.0229) (-9.2272, 11.0365) (-9.2918, 11.0496) (-9.3566, 11.0623) (-9.4216, 11.0746) (-9.4869, 11.0864) (-9.5524, 11.0978) (-9.6182, 11.1087) (-9.6841, 11.1192) (-9.7503, 11.1292) (-9.8167, 11.1388) (-9.8833, 11.148) (-9.9368, 11.155) (-9.977, 11.16) (-10.0038, 11.1633) (-10.0173, 11.1649) knots 0 0 0 0 0 0 0.01428571 0.02857143 0.04285714 0.05714286 0.07142857 0.08571429 0.1 0.11428571 0.12857143 0.14285714 0.15714286 0.17142857 0.18571429 0.2 0.21428571 0.22857143 0.24285714 0.25714286 0.27142857 0.28571429 0.3 0.31428571 0.32857143 0.34285714 0.35714286 0.37142857 0.38571429 0.4 0.41428571 0.42857143 0.44285714 0.45714286 0.47142857 0.48571429 0.5 0.51428571 0.52857143 0.54285714 0.55714286 0.57142857 0.58571429 0.6 0.61428571 0.62857143 0.64285714 0.65714286 0.67142857 0.68571429 0.7 0.71428571 0.72857143 0.74285714 0.75714286 0.77142857 0.78571429 0.8 0.81428571 0.82857143 0.84285714 0.85714286 0.87142857 0.88571429 0.9 0.91428571 0.92857143 0.94285714 0.95714286 0.97142857 0.98571429 1 1 1 1 1 1
  arc A23 (-10.0173, 11.1649) -> (-11.1649, 10.0173) centre (0, 0) ccw
  spline S15 degree 5 poles (-11.1649, 10.0173) (-11.1633, 10.0038) (-11.16, 9.977) (-11.155, 9.9368) (-11.148, 9.8833) (-11.1388, 9.8167) (-11.1292, 9.7503) (-11.1192, 9.6841) (-11.1087, 9.6182) (-11.0978, 9.5524) (-11.0864, 9.4869) (-11.0746, 9.4216) (-11.0623, 9.3566) (-11.0496, 9.2918) (-11.0365, 9.2272) (-11.0229, 9.1629) (-11.0089, 9.0989) (-10.9944, 9.0351) (-10.9795, 8.9716) (-10.9641, 8.9083) (-10.9483, 8.8454) (-10.9321, 8.7826) (-10.9154, 8.7202) (-10.8983, 8.6581) (-10.8807, 8.5962) (-10.8626, 8.5347) (-10.8442, 8.4734) (-10.8252, 8.4125) (-10.8059, 8.3519) (-10.7861, 8.2915) (-10.7658, 8.2315) (-10.7451, 8.1719) (-10.7239, 8.1125) (-10.7023, 8.0535) (-10.6802, 7.9949) (-10.6576, 7.9366) (-10.6346, 7.8786) (-10.6112, 7.821) (-10.5873, 7.7638) (-10.5629, 7.707) (-10.5381, 7.6505) (-10.5128, 7.5944) (-10.4871, 7.5388) (-10.4608, 7.4835) (-10.4341, 7.4287) (-10.407, 7.3743) (-10.3793, 7.3203) (-10.3512, 7.2667) (-10.3226, 7.2136) (-10.2936, 7.1609) (-10.264, 7.1088) (-10.234, 7.0571) (-10.2034, 7.0059) (-10.1723, 6.9553) (-10.1406, 6.9053) (-10.1085, 6.8557) (-10.0759, 6.8067) (-10.0428, 6.7581) (-10.0092, 6.7101) (-9.9752, 6.6626) (-9.9405, 6.6158) (-9.9051, 6.5698) (-9.869, 6.5248) (-9.8321, 6.4806) (-9.7945, 6.4373) (-9.7564, 6.3946) (-9.718, 6.3524) (-9.6792, 6.3106) (-9.6399, 6.2695) (-9.5998, 6.2295) (-9.5583, 6.1913) (-9.5235, 6.1629) (-9.4963, 6.1431) (-9.4777, 6.1305) (-9.4682, 6.1244) knots -1 -1 -1 -1 -1 -1 -0.98571429 -0.97142857 -0.95714286 -0.94285714 -0.92857143 -0.91428571 -0.9 -0.88571429 -0.87142857 -0.85714286 -0.84285714 -0.82857143 -0.81428571 -0.8 -0.78571429 -0.77142857 -0.75714286 -0.74285714 -0.72857143 -0.71428571 -0.7 -0.68571429 -0.67142857 -0.65714286 -0.64285714 -0.62857143 -0.61428571 -0.6 -0.58571429 -0.57142857 -0.55714286 -0.54285714 -0.52857143 -0.51428571 -0.5 -0.48571429 -0.47142857 -0.45714286 -0.44285714 -0.42857143 -0.41428571 -0.4 -0.38571429 -0.37142857 -0.35714286 -0.34285714 -0.32857143 -0.31428571 -0.3 -0.28571429 -0.27142857 -0.25714286 -0.24285714 -0.22857143 -0.21428571 -0.2 -0.18571429 -0.17142857 -0.15714286 -0.14285714 -0.12857143 -0.11428571 -0.1 -0.08571429 -0.07142857 -0.05714286 -0.04285714 -0.02857143 -0.01428571 0 0 0 0 0 0
  line L15 (-9.4682, 6.1244) -> (-8.2357, 5.3259)
  arc A24 (-7.6452, 3.3555) -> (-8.2357, 5.3259) centre (-9.0989, 3.9936) ccw
  arc A25 (1.5106, -1.992) -> (-1.5106, -1.992) centre (0, 0) ccw
  line L16 (0, -1.992) -> (-1.5106, -1.992)
  line L17 (1.5106, -1.992) -> (0, -1.992)
  line L18 (0, -2.092) -> (-1.5439, -2.092)
  arc A26 (1.5439, -2.092) -> (-1.5439, -2.092) centre (0, 0) ccw
  line L19 (1.5439, -2.092) -> (0, -2.092)
  arc A27 (-7.7787, -3.0333) -> (-7.6452, -3.3555) centre (0, 0) ccw
  arc A28 (-3.3555, -7.6452) -> (-3.0333, -7.7787) centre (0, 0) ccw
  arc A29 (3.0333, -7.7787) -> (3.3555, -7.6452) centre (0, 0) ccw
  arc A30 (7.6452, -3.3555) -> (7.7787, -3.0333) centre (0, 0) ccw
  arc A31 (7.7787, 3.0333) -> (7.6452, 3.3555) centre (0, 0) ccw
  arc A32 (3.3555, 7.6452) -> (3.0333, 7.7787) centre (0, 0) ccw
  arc A33 (-3.0333, 7.7787) -> (-3.3555, 7.6452) centre (0, 0) ccw
  dimension "d10" = 0.1
extrude "Extrude3" cut sketch "Sketch1 (2)" against normal through all contours A25 L16 L17 | L18 A26 L19 bodies 2 in component "Spur Gear (8 teeth)"
component "Spur Gear (8 teeth)" placed x (1, 0, 0) y (0, 1, 0) z (0, 0, 1) at (0, 0, 0)
hidden bodies 1
equation "pmma_thickness_Ref = 10 mm" comment "The thickness of the Perspex (Poly Methyl Meth Acrylaat) plate"
equation "d2 = pmma_thickness_Ref"
equation "d4 = pmma_thickness_Ref"
equation "rotate_motor_Ref = 117 deg"
named bodies: "Body6"
